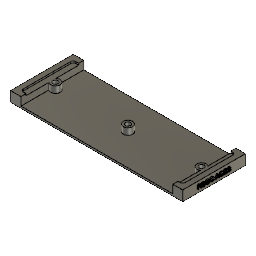
FullSizeHolder v4 (Autodesk Fusion 360 design; units mm, degrees)
Autodesk Fusion 360 part; units mm, degrees
sketch "Solid" plane through (0, 0, 0) normal (0, 0, 1) x (1, 0, 0)
  line L0 (83.5, -30.5) -> (-83.5, -30.5)
  line L1 (-83.5, -30.5) -> (-83.5, 30.5)
  line L2 (-83.5, 30.5) -> (83.5, 30.5)
  line L3 (83.5, 30.5) -> (83.5, -30.5)
  line L4 (83.5, -30.5) -> (-83.5, 30.5) construction
  line L5 (-83.5, -30.5) -> (83.5, 30.5) construction
  dimension "d13" = 167
  dimension "d14" = 61
  constraint horizontal L0
  constraint perpendicular L0 L1
  constraint parallel L0 L2
  constraint parallel L1 L3
  constraint coincident L4 origin
  constraint coincident L5 origin
  measures "d13" distance of L1.end L2.end
  measures "d14" distance of L0.end L1.end
extrude "Extrude1" add sketch "Solid" along normal blind 10
sketch "FR4Recess" plane through (0, 0, 10) normal (0, 0, 1) x (-1, 0, 0)
  line L0 (-83.5, -30.5) -> (83.5, -30.5)
  line L1 (83.5, -30.5) -> (83.5, 30.5)
  line L2 (83.5, 30.5) -> (-83.5, 30.5)
  line L3 (-83.5, 30.5) -> (-83.5, -30.5)
  line L4 (75.96, 25.5) -> (-75.96, 25.5)
  line L5 (-78.5, 22.96) -> (-78.5, -22.96)
  line L6 (-75.96, -25.5) -> (75.96, -25.5)
  line L7 (78.5, -22.96) -> (78.5, 22.96)
  line L8 (78.5, 25.5) -> (-78.5, -25.5) construction
  line L9 (-78.5, 25.5) -> (78.5, -25.5) construction
  arc A0 (75.96, -25.5) -> (78.5, -22.96) centre (75.96, -22.96) ccw
  arc A1 (78.5, 22.96) -> (75.96, 25.5) centre (75.96, 22.96) ccw
  arc A2 (-75.96, 25.5) -> (-78.5, 22.96) centre (-75.96, 22.96) ccw
  arc A3 (-78.5, -22.96) -> (-75.96, -25.5) centre (-75.96, -22.96) ccw
  dimension "d17" = 157
  dimension "d18" = 51
  dimension "d19" = 2.54
  dimension "d20" = 2.54
  dimension "d21" = 2.54
  dimension "d22" = 2.54
  constraint horizontal L4
  constraint perpendicular L4 L5
  constraint parallel L4 L6
  constraint parallel L5 L7
  constraint coincident L8 origin
  constraint coincident L9 origin
  constraint coincident L9.end L6
  constraint coincident L9.end L7
  constraint tangent L6 A0
  constraint tangent L7 A0
  constraint coincident L8.start L4
  constraint coincident L8.start L7
  constraint tangent L4 A1
  constraint tangent L7 A1
  constraint coincident L9.start L4
  constraint coincident L9.start L5
  constraint tangent L4 A2
  constraint tangent L5 A2
  constraint coincident L8.end L6
  constraint coincident L8.end L5
  constraint tangent L6 A3
  constraint tangent L5 A3
  measures "d17" distance of L8.end L9.end
  measures "d18" distance of L9.start L8.end
  measures "d19" radius of A0
  measures "d20" radius of A1
  measures "d21" radius of A2
  measures "d22" radius of A3
extrude "Extrude2" cut sketch "FR4Recess" against normal blind 1.68 contours L4 L5 L6 L7 A0 A1 A2 A3
sketch "Extrude" plane through (0, 0, 10) normal (0, 0, 1) x (-1, 0, 0)
  line L0 (73.2312, -31.7537) -> (-73.9375, -31.7537)
  line L1 (-73.9375, -31.7537) -> (-73.9375, 32.0704)
  line L2 (-73.9375, 32.0704) -> (73.2312, 32.0704)
  line L3 (73.2312, 32.0704) -> (73.2312, -31.7537)
  constraint horizontal L0
  constraint vertical L1
  constraint horizontal L2
  constraint vertical L3
extrude "Extrude6" cut sketch "Extrude" against normal blind 8
sketch "PierCenter" plane through (0, 0, 2) normal (0, 0, 1) x (-1, 0, 0)
  line L0 (73.2312, 30.5) -> (-73.9375, 30.5)
  line L1 (-73.9375, 30.5) -> (-73.9375, -30.5)
  line L2 (-73.9375, -30.5) -> (73.2312, -30.5)
  line L3 (73.2312, -30.5) -> (73.2312, 30.5)
  circle A0 centre (0, 0) radius 4.5
  circle A1 centre (0, 0) radius 2.5
  dimension "d33" = 9
  dimension "d34" = 5
  constraint coincident A0.centre A1.centre
  constraint concentric A0 A1
  measures "d33" diameter of A0
  measures "d34" diameter of A1
extrude "Extrude7" add sketch "PierCenter" along normal blind 6.32 contours A0
sketch "PierLeft" plane through (0, 0, 2) normal (0, 0, 1) x (-1, 0, 0)
  line L0 (73.2312, 30.5) -> (-73.9375, 30.5)
  line L1 (-73.9375, 30.5) -> (-73.9375, -30.5)
  line L2 (-73.9375, -30.5) -> (73.2312, -30.5)
  line L3 (73.2312, -30.5) -> (73.2312, 30.5)
  circle A0 centre (0, 0) radius 4.5
  circle A1 centre (70.3114, -0.0182) radius 4.5
  circle A2 centre (70.3114, -0.0182) radius 2.5
  point P0 (70.3114, -0.0182)
  dimension "d37" = 9
  dimension "d38" = 5
  constraint coincident P0 A1.centre
  measures "d37" diameter of A1
  measures "d38" diameter of A2
extrude "Extrude8" add sketch "PierLeft" along normal blind 6.32 contours L3 A1 picked at (66.4862, -0.0182)
sketch "PierRight" plane through (0, 0, 2) normal (0, 0, 1) x (-1, 0, 0)
  arc A0 (73.2312, 3.406) -> (73.2312, -3.4424) centre (70.3114, -0.0182) ccw
  line L0 (73.2312, 3.406) -> (73.2312, 30.5)
  line L1 (73.2312, 30.5) -> (-73.9375, 30.5)
  line L2 (-73.9375, 30.5) -> (-73.9375, -30.5)
  line L3 (-73.9375, -30.5) -> (73.2312, -30.5)
  line L4 (73.2312, -30.5) -> (73.2312, -3.4424)
  circle A1 centre (0, 0) radius 4.5
  circle A2 centre (-71.2906, 0.0558) radius 4.5
  circle A3 centre (-71.2906, 0.0558) radius 2.5
  point P0 (-71.2906, 0.0558)
  dimension "d41" = 9
  dimension "d42" = 5
  constraint coincident P0 A2.centre
  constraint concentric A2 A3
  measures "d41" diameter of A2
  measures "d42" diameter of A3
extrude "Extrude9" add sketch "PierRight" along normal blind 6.32 contours L2 A2 picked at (-73.2852, 3.3195)
sketch "RSGCACES" plane through (83.5, 0, 0) normal (1, 0, 0) x (0, 1, 0)
  line L0 (-30.5, 0) -> (30.5, 0)
  line L1 (30.5, 0) -> (30.5, 10)
  line L2 (30.5, 10) -> (-30.5, 10)
  line L3 (-30.5, 10) -> (-30.5, 0)
  line L4 (-18.8418, 2.2772) -> (17.8909, 2.2772) construction
  line L5 (17.8909, 2.2772) -> (17.8909, 8.5407) construction
  line L6 (17.8909, 8.5407) -> (-18.8418, 8.5407) construction
  line L7 (-18.8418, 8.5407) -> (-18.8418, 2.2772) construction
  dimension "d45" = 4
  text T0 "RSGC ACES" font "Arial" height 4 align centre middle in box 36.7327 x 6.2635 at (-18.8418, 2.2772) x (1, 0) y (0, 1) spacing 1 kerned
extrude "Extrude10" add sketch "RSGCACES" along normal blind 1 text T0
sketch "PermaProto" plane through (-83.5, 0, 0) normal (-1, 0, 0) x (0, -1, 0)
  line L0 (-30.5, 0) -> (30.5, 0)
  line L1 (30.5, 0) -> (30.5, 10)
  line L2 (30.5, 10) -> (-30.5, 10)
  line L3 (-30.5, 10) -> (-30.5, 0)
  line L4 (-23.5941, 1.9572) -> (24.0905, 1.9572) construction
  line L5 (24.0905, 1.9572) -> (24.0905, 8.5295) construction
  line L6 (24.0905, 8.5295) -> (-23.5941, 8.5295) construction
  line L7 (-23.5941, 8.5295) -> (-23.5941, 1.9572) construction
  dimension "d48" = 4
  text T0 "Perma-Proto" font "Arial" height 4 align centre middle in box 47.6846 x 6.5724 at (-23.5941, 1.9572) x (1, 0) y (0, 1) spacing 1 kerned
extrude "Extrude11" add sketch "PermaProto" along normal blind 1 text T0
sketch "ACESLogo" plane through (0, 0, 0) normal (0, 0, 1) x (1, 0, 0)
  arc A0 (-0.5552, -1.4875) -> (-1.5641, -1.6462) centre (-1.6183, 1.9835) cw
  spline S0 degree 3 poles (-1.5641, -1.6462) (-2.3665, -1.5998) (-3.0241, -0.9925) (-3.134, -0.1963) knots 1 1 1 1 2 2 2 2
  arc A1 (-3.134, -0.1963) -> (-2.6789, 1.1936) centre (-1.2347, -0.0487) cw
  spline S1 degree 3 poles (-2.6789, 1.1936) (-1.9451, 2.0932) (-1.2008, 2.9857) (-0.467, 3.8889) knots 3 3 3 3 4 4 4 4
  spline S2 degree 3 poles (-0.467, 3.8889) (-0.307, 4.097) (-0.0088, 4.1364) (0.1997, 3.9771) knots 4 4 4 4 5 5 5 5
  arc A2 (0.1997, 3.9771) -> (0.2879, 3.8889) centre (-0.0472, 3.6419) cw
  spline S3 degree 3 poles (0.2879, 3.8889) (0.7289, 3.3279) (1.1981, 2.7952) (1.6497, 2.2449) knots 6 6 6 6 7 7 7 7
  arc A3 (1.6497, 2.2449) -> (2.6657, 0.982) centre (-8.6979, -7.1195) cw
  spline S4 degree 3 poles (2.6657, 0.982) (3.195, 0.2422) (3.0262, -0.7863) (2.2882, -1.3181) knots 8 8 8 8 9 9 9 9
  arc A4 (2.2882, -1.3181) -> (1.7026, -1.5827) centre (1.3109, 0.0647) cw
  arc A5 (1.7026, -1.5827) -> (0.5702, -1.5263) centre (1.2508, 0.7409) cw
  spline S5 degree 3 poles (0.5702, -1.5263) (0.5067, -1.5263) (0.422, -1.4451) (0.3373, -1.551) (0.4044, -1.6251) (0.4255, -1.6886) knots 11 11 11 11 12 12 13 13 13 13
  arc A6 (0.4255, -1.6886) -> (0.7889, -2.3341) centre (4.0074, -0.0976) ccw
  spline S6 degree 3 poles (0.7889, -2.3341) (0.8348, -2.4047) (0.8947, -2.4788) (0.7889, -2.6622) (0.7007, -2.6446) (0.6125, -2.6446) knots 14 14 14 14 15 15 16 16 16 16
  line L0 (0.6125, -2.6446) -> (-0.7986, -2.6446)
  arc A7 (-0.7986, -2.6446) -> (-0.9785, -2.5634) centre (-0.8165, -2.4443) cw
  spline S7 degree 3 poles (-0.9785, -2.5634) (-1.0279, -2.4894) (-0.9785, -2.4294) (-0.9503, -2.3694) knots 18 18 18 18 19 19 19 19
  arc A8 (-0.9503, -2.3694) -> (-0.5552, -1.4875) centre (-3.2707, -0.8004) ccw
  arc A9 (0.362, -5.6326) -> (0.7501, -6.4899) centre (3.1563, -4.8842) ccw
  arc A10 (0.7501, -6.4899) -> (0.8171, -6.5886) centre (-0.0176, -7.0829) cw
  spline S8 degree 3 poles (0.8171, -6.5886) (0.8585, -6.657) (0.8367, -6.7459) (0.7684, -6.7873) knots 2 2 2 2 3 3 3 3
  spline S9 degree 3 poles (0.7684, -6.7873) (0.767, -6.7881) (0.7656, -6.7889) (0.7642, -6.7897) knots 3 3 3 3 4 4 4 4
  arc A11 (0.7642, -6.7897) -> (0.6795, -6.8109) centre (0.6938, -6.6882) cw
  line L1 (0.6795, -6.8109) -> (-0.8692, -6.8109)
  spline S10 degree 3 poles (-0.8692, -6.8109) (-1.0138, -6.8109) (-1.0703, -6.698) (-0.9926, -6.571) knots 6 6 6 6 7 7 7 7
  arc A12 (-0.9926, -6.571) -> (-0.5975, -5.7984) centre (-4.0766, -4.5065) ccw
  spline S11 degree 3 poles (-0.5975, -5.7984) (-0.5799, -5.749) (-0.5481, -5.6926) (-0.6469, -5.622) (-0.6787, -5.6573) (-0.721, -5.6785) knots 8 8 8 8 9 9 10 10 10 10
  arc A13 (-0.721, -5.6785) -> (-2.1533, -5.6573) centre (-1.4054, -3.5232) cw
  spline S12 degree 3 poles (-2.1533, -5.6573) (-2.7471, -5.4029) (-3.1374, -4.825) (-3.1516, -4.1792) knots 11 11 11 11 12 12 12 12
  arc A14 (-3.1516, -4.1792) -> (-3.0917, -3.6923) centre (-1.2679, -4.1641) cw
  spline S13 degree 3 poles (-3.0917, -3.6923) (-3.0773, -3.6102) (-3.0018, -3.5531) (-2.9188, -3.5618) knots 13 13 13 13 14 14 14 14
  line L2 (-2.9188, -3.5618) -> (2.6445, -3.5618)
  spline S14 degree 3 poles (2.6445, -3.5618) (2.8032, -3.5618) (2.8738, -3.6147) (2.9056, -3.7594) knots 15 15 15 15 16 16 16 16
  spline S15 degree 3 poles (2.9056, -3.7594) (3.1249, -4.6304) (2.5966, -5.5142) (1.7256, -5.7336) knots 16 16 16 16 17 17 17 17
  line L3 (1.7256, -5.7336) -> (1.7202, -5.7349)
  line L4 (1.7202, -5.7349) -> (1.6673, -5.7349)
  arc A15 (1.6673, -5.7349) -> (0.362, -5.6326) centre (1.2187, -3.0809) cw
  spline S16 degree 3 poles (-4.9861, -1.4875) (-5.2154, -1.5439) (-5.4341, -1.5898) (-5.6528, -1.6251) knots 0 0 0 0 1 1 1 1
  spline S17 degree 3 poles (-5.6528, -1.6251) (-6.5586, -1.7725) (-7.4123, -1.1577) (-7.5598, -0.252) (-7.6373, 0.2242) (-7.5039, 0.7106) (-7.1945, 1.0808) knots 1 1 1 1 2 2 2 3 3 3 3
  spline S18 degree 3 poles (-7.1945, 1.0808) (-6.7606, 1.6417) (-6.2984, 2.1779) (-5.8539, 2.7247) knots 3 3 3 3 4 4 4 4
  line L5 (-5.8539, 2.7247) -> (-4.8944, 3.8959)
  arc A16 (-4.8944, 3.8959) -> (-4.5416, 4.0723) centre (-4.5522, 3.6526) cw
  spline S19 degree 3 poles (-4.5416, 4.0723) (-4.454, 4.0763) (-4.3798, 4.0085) (-4.3758, 3.9209) knots 6 6 6 6 7 7 7 7
  line L6 (-4.3758, 3.9209) -> (-4.3758, 3.9206)
  line L7 (-4.3758, 3.9206) -> (-4.3758, -2.4858)
  spline S20 degree 3 poles (-4.3758, -2.4858) (-4.356, -2.5763) (-4.4126, -2.6659) (-4.5028, -2.6869) knots 9 9 9 9 10 10 10 10
  line L8 (-4.5028, -2.6869) -> (-5.2577, -2.6869)
  arc A17 (-5.2577, -2.6869) -> (-5.4482, -2.5917) centre (-5.2823, -2.498) cw
  spline S21 degree 3 poles (-5.4482, -2.5917) (-5.4941, -2.5246) (-5.4482, -2.4682) (-5.4129, -2.4153) knots 12 12 12 12 13 13 13 13
  arc A18 (-5.4129, -2.4153) -> (-4.9861, -1.4875) centre (-7.9879, -0.6685) ccw
  line L9 (4.2002, 0.7068) -> (4.2002, 3.8077)
  spline S22 degree 3 poles (4.2002, 3.8077) (4.2002, 3.8994) (4.1614, 4.0159) (4.2814, 4.0582) knots 1 1 1 1 2 2 2 2
  arc A19 (4.2814, 4.0582) -> (4.6059, 3.9876) centre (4.3827, 3.7424) cw
  arc A20 (4.6059, 3.9876) -> (4.9305, 3.6102) centre (2.8461, 2.1463) cw
  spline S23 degree 3 poles (4.9305, 3.6102) (5.6184, 2.7811) (6.3169, 1.9556) (6.9837, 1.109) knots 4 4 4 4 5 5 5 5
  spline S24 degree 3 poles (6.9837, 1.109) (7.5909, 0.4209) (7.5253, -0.6291) (6.8372, -1.2363) (6.4609, -1.5684) (5.9545, -1.7126) (5.4597, -1.6286) knots 5 5 5 5 6 6 6 7 7 7 7
  spline S25 degree 3 poles (5.4597, -1.6286) (5.2692, -1.6004) (5.0857, -1.5686) (4.8988, -1.5228) knots 7 7 7 7 8 8 8 8
  spline S26 degree 3 poles (4.8988, -1.5228) (4.8705, -1.5228) (4.8458, -1.4839) (4.7894, -1.5616) (4.8176, -1.5757) (4.8176, -1.6074) knots 8 8 8 8 9 9 10 10 10 10
  arc A21 (4.8176, -1.6074) -> (5.1457, -2.313) centre (7.942, -0.5836) ccw
  spline S27 degree 3 poles (5.1457, -2.313) (5.2021, -2.4118) (5.315, -2.5035) (5.181, -2.7504) (5.0399, -2.6975) (4.9305, -2.701) knots 11 11 11 11 12 12 13 13 13 13
  line L10 (4.9305, -2.701) -> (4.4013, -2.701)
  spline S28 degree 3 poles (4.4013, -2.701) (4.2249, -2.701) (4.1967, -2.6658) (4.1967, -2.4999) knots 14 14 14 14 15 15 15 15
  line L11 (4.1967, -2.4999) -> (4.2002, 0.7068)
  line L12 (2.3023, 5.0036) -> (0.9723, 5.0036)
  spline S29 degree 3 poles (0.9723, 5.0036) (0.4679, 5.0036) (-0.0401, 4.9789) (-0.5446, 5.0036) knots 1 1 1 1 2 2 2 2
  line L13 (-0.5446, 5.0036) -> (-2.6048, 5.0036)
  arc A22 (-2.6048, 5.0036) -> (-2.7777, 5.0918) centre (-2.6224, 5.1827) cw
  ellipse E0 centre (-2.6432, 5.157) end of major axis (-2.6115, 5.304) minor radius 0.1488 (-2.7389, 5.2717) -> (-2.7777, 5.0918) ccw
  arc A23 (-2.7389, 5.2717) -> (-0.467, 8.0305) centre (494.7406, -402.1025) cw
  spline S30 degree 3 poles (-0.467, 8.0305) (-0.3293, 8.2375) (-0.0502, 8.2943) (0.1574, 8.1575) knots 6 6 6 6 7 7 7 7
  arc A24 (0.1574, 8.1575) -> (0.2985, 8.0093) centre (-0.08, 7.7901) cw
  spline S31 degree 3 poles (0.2985, 8.0093) (0.6125, 7.6177) (0.9406, 7.2367) (1.2616, 6.8487) knots 8 8 8 8 9 9 9 9
  line L14 (1.2616, 6.8487) -> (2.3199, 5.554)
  spline S32 degree 3 poles (2.3199, 5.554) (2.3976, 5.4587) (2.4716, 5.3635) (2.5528, 5.2753) knots 10 10 10 10 11 11 11 11
  ellipse E1 centre (2.4602, 5.1624) end of major axis (2.4286, 5.3059) minor radius 0.1453 (2.5916, 5.0989) -> (2.5528, 5.2753) ccw
  spline S33 degree 3 poles (2.5916, 5.0989) (2.5643, 5.0318) (2.4934, 4.9934) (2.4223, 5.0072) knots 12 12 12 12 13 13 13 13
  arc A25 (2.4223, 5.0072) -> (2.3023, 5.0036) centre (2.3725, 4.6579) ccw
  arc A26 (4.8423, -5.6397) -> (5.248, -6.5004) centre (7.9138, -4.718) ccw
  spline S34 degree 3 poles (5.248, -6.5004) (5.2903, -6.5675) (5.3397, -6.631) (5.248, -6.8074) (5.1669, -6.7862) (5.0963, -6.7862) knots 1 1 1 1 2 2 3 3 3 3
  line L15 (5.0963, -6.7862) -> (4.419, -6.7862)
  spline S35 degree 3 poles (4.419, -6.7862) (4.2849, -6.7862) (4.232, -6.7297) (4.232, -6.5957) knots 4 4 4 4 5 5 5 5
  line L16 (4.232, -6.5957) -> (4.232, -3.7453)
  spline S36 degree 3 poles (4.232, -3.7453) (4.232, -3.6147) (4.2884, -3.5477) (4.419, -3.5477) knots 6 6 6 6 7 7 7 7
  line L17 (4.419, -3.5477) -> (7.1848, -3.5477)
  spline S37 degree 3 poles (7.1848, -3.5477) (7.2676, -3.5364) (7.3454, -3.5898) (7.3647, -3.6712) knots 8 8 8 8 9 9 9 9
  spline S38 degree 3 poles (7.3647, -3.6712) (7.6112, -4.543) (7.1043, -5.4495) (6.2325, -5.696) knots 9 9 9 9 10 10 10 10
  line L18 (6.2325, -5.696) -> (6.2323, -5.6961)
  arc A27 (6.2323, -5.6961) -> (6.0029, -5.742) centre (5.7724, -3.9931) cw
  arc A28 (6.0029, -5.742) -> (4.9446, -5.622) centre (5.7859, -2.9281) cw
  line L19 (4.9446, -5.622) -> (4.8846, -5.622)
  line L20 (4.8846, -5.622) -> (4.8423, -5.6397)
  arc A29 (-4.9896, -5.6361) -> (-5.9774, -5.7808) centre (-6.0199, -2.0451) cw
  spline S39 degree 3 poles (-5.9774, -5.7808) (-6.5657, -5.7727) (-7.1045, -5.4494) (-7.3885, -4.9341) knots 1 1 1 1 2 2 2 2
  arc A30 (-7.3885, -4.9341) -> (-7.5331, -3.7453) centre (-6.0354, -4.1663) cw
  spline S40 degree 3 poles (-7.5331, -3.7453) (-7.5138, -3.6474) (-7.4245, -3.5793) (-7.325, -3.5865) knots 3 3 3 3 4 4 4 4
  line L21 (-7.325, -3.5865) -> (-4.6051, -3.5865)
  spline S41 degree 3 poles (-4.6051, -3.5865) (-4.4252, -3.5865) (-4.3934, -3.6253) (-4.3934, -3.8123) knots 5 5 5 5 6 6 6 6
  line L22 (-4.3934, -3.8123) -> (-4.3934, -6.6027)
  spline S42 degree 3 poles (-4.3934, -6.6027) (-4.3934, -6.7544) (-4.4428, -6.8109) (-4.598, -6.8109) knots 7 7 7 7 8 8 8 8
  line L23 (-4.598, -6.8109) -> (-5.2507, -6.8109)
  arc A31 (-5.2507, -6.8109) -> (-5.4482, -6.7297) centre (-5.2863, -6.6166) cw
  spline S43 degree 3 poles (-5.4482, -6.7297) (-5.4976, -6.6486) (-5.4482, -6.5957) (-5.4094, -6.5357) knots 10 10 10 10 11 11 11 11
  arc A32 (-5.4094, -6.5357) -> (-4.9896, -5.6361) centre (-7.8372, -4.855) ccw
  line L24 (4.2285, 6.5982) -> (4.2285, 8.0093)
  spline S44 degree 3 poles (4.2285, 8.0093) (4.2285, 8.1963) (4.3167, 8.2739) (4.5248, 8.2139) knots 1 1 1 1 2 2 2 2
  arc A33 (4.5248, 8.2139) -> (4.7329, 8.0728) centre (4.402, 7.8088) cw
  line L25 (4.7329, 8.0728) -> (5.7913, 6.7746)
  line L26 (5.7913, 6.7746) -> (6.9696, 5.3635)
  arc A34 (6.9696, 5.3635) -> (7.0613, 5.2435) centre (6.5428, 4.9421) cw
  spline S45 degree 3 poles (7.0613, 5.2435) (7.1007, 5.1832) (7.0837, 5.1023) (7.0234, 5.0629) knots 6 6 6 6 7 7 7 7
  ellipse E2 centre (6.9292, 5.1661) end of major axis (7.0726, 5.1299) minor radius 0.1252 (7.0189, 5.0601) -> (7.0234, 5.0629) ccw
  arc A35 (7.0189, 5.0601) -> (6.9449, 5.0389) centre (6.9426, 5.1871) cw
  line L27 (6.9449, 5.0389) -> (4.3625, 5.0389)
  spline S46 degree 3 poles (4.3625, 5.0389) (4.2355, 5.0389) (4.2249, 5.1271) (4.2249, 5.2259) knots 10 10 10 10 11 11 11 11
  line L28 (4.2249, 5.2259) -> (4.2249, 6.5982)
  line L29 (4.2249, 6.5982) -> (4.2285, 6.5982)
  spline S47 degree 3 poles (-4.404, 6.958) (-4.3722, 6.5559) (-4.4216, 6.0796) (-4.3828, 5.6069) knots 0 0 0 0 1 1 1 1
  line L30 (-4.3828, 5.6069) -> (-4.3828, 5.1589)
  spline S48 degree 3 poles (-4.3828, 5.1589) (-4.3768, 5.0753) (-4.4396, 5.0027) (-4.5232, 4.9966) knots 2 2 2 2 3 3 3 3
  line L31 (-4.5232, 4.9966) -> (-4.5239, 4.9966)
  line L32 (-4.5239, 4.9966) -> (-6.1326, 4.9966)
  line L33 (-6.1326, 4.9966) -> (-7.0851, 4.9966)
  spline S49 degree 3 poles (-7.0851, 4.9966) (-7.1607, 4.9884) (-7.2285, 5.0431) (-7.2367, 5.1186) knots 6 6 6 6 7 7 7 7
  line L34 (-7.2367, 5.1186) -> (-7.2368, 5.1201)
  arc A36 (-7.2368, 5.1201) -> (-7.1909, 5.2365) centre (-7.0925, 5.1305) cw
  spline S50 degree 3 poles (-7.1909, 5.2365) (-6.8382, 5.6633) (-6.4854, 6.0902) (-6.1326, 6.51) knots 9 9 9 9 10 10 10 10
  line L35 (-6.1326, 6.51) -> (-5.2083, 7.6989)
  spline S51 degree 3 poles (-5.2083, 7.6989) (-5.106, 7.8259) (-5.0002, 7.9564) (-4.8944, 8.0799) knots 11 11 11 11 12 12 12 12
  arc A37 (-4.8944, 8.0799) -> (-4.591, 8.221) centre (-4.5754, 7.7909) cw
  spline S52 degree 3 poles (-4.591, 8.221) (-4.5059, 8.2316) (-4.4283, 8.1713) (-4.4177, 8.0862) (-4.416, 8.0724) (-4.4161, 8.0584) (-4.4181, 8.0446) knots 13 13 13 13 14 14 14 15 15 15 15
  spline S53 degree 3 poles (-4.4181, 8.0446) (-4.4075, 7.7059) (-4.404, 7.3672) (-4.404, 6.958) knots 15 15 15 15 16 16 16 16
  line L36 (8.2784, 0.1565) -> (8.2784, 1.6276)
  spline S54 degree 3 poles (8.2784, 1.6276) (8.2784, 1.7087) (8.2784, 1.7863) (8.3666, 1.8181) knots 1 1 1 1 2 2 2 2
  spline S55 degree 3 poles (8.3666, 1.8181) (8.4344, 1.8499) (8.5153, 1.8274) (8.5571, 1.7651) knots 2 2 2 2 3 3 3 3
  spline S56 degree 3 poles (8.5571, 1.7651) (8.7617, 1.4935) (9.0121, 1.2536) (9.1921, 0.9608) knots 3 3 3 3 4 4 4 4
  spline S57 degree 3 poles (9.1921, 0.9608) (9.5878, 0.3976) (9.5962, -0.3511) (9.2132, -0.923) knots 4 4 4 4 5 5 5 5
  arc A38 (9.2132, -0.923) -> (8.55, -1.4804) centre (7.7815, 0.1073) cw
  spline S58 degree 3 poles (8.55, -1.4804) (8.3736, -1.5721) (8.2713, -1.5016) (8.2713, -1.3005) knots 6 6 6 6 7 7 7 7
  line L37 (8.2713, -1.3005) -> (8.2713, 0.1565)
  line L38 (8.2713, 0.1565) -> (8.2784, 0.1565)
  line L39 (-8.4786, 0.1353) -> (-8.4786, -1.3111)
  ellipse E3 centre (-9.7979, 0.5867) end of major axis (-11.0461, 2.6795) minor radius 0.4973 (-8.7467, -1.4804) -> (-8.4786, -1.3111) ccw
  spline S59 degree 3 poles (-8.7467, -1.4804) (-9.2238, -1.2603) (-9.5645, -0.8223) (-9.6604, -0.3057) knots 2 2 2 2 3 3 3 3
  ellipse E4 centre (-7.9359, -0.0084) end of major axis (-7.4669, 1.6844) minor radius 1.7485 (-9.2617, 1.1337) -> (-9.6604, -0.3057) ccw
  spline S60 degree 3 poles (-9.2617, 1.1337) (-9.0889, 1.3489) (-8.9196, 1.5464) (-8.7361, 1.7722) knots 4 4 4 4 5 5 5 5
  ellipse E5 centre (-8.6173, 1.6875) end of major axis (-8.4758, 1.7271) minor radius 0.1453 (-8.5597, 1.8216) -> (-8.7361, 1.7722) ccw
  spline S61 degree 3 poles (-8.5597, 1.8216) (-8.4821, 1.7934) (-8.4645, 1.7334) (-8.4645, 1.6558) knots 6 6 6 6 7 7 7 7
  spline S62 degree 3 poles (-8.4645, 1.6558) (-8.4821, 1.1513) (-8.4786, 0.6504) (-8.4786, 0.1353) knots 7 7 7 7 8 8 8 8
  line L40 (-0.1036, 9.0888) -> (-1.162, 9.0888)
  spline S63 degree 3 poles (-1.162, 9.0888) (-1.2431, 9.0888) (-1.3137, 9.0888) (-1.3913, 9.2723) (-1.3525, 9.3146) (-1.296, 9.371) knots 1 1 1 1 2 2 3 3 3 3
  line L41 (-1.296, 9.371) -> (-0.4353, 10.4294)
  spline S64 degree 3 poles (-0.4353, 10.4294) (-0.2676, 10.6162) (0.0197, 10.632) (0.2068, 10.4646) knots 4 4 4 4 5 5 5 5
  ellipse E6 centre (-0.0094, 10.2133) end of major axis (0.3199, 10.1741) minor radius 0.3315 (0.2421, 10.4294) -> (0.2068, 10.4646) ccw
  spline S65 degree 3 poles (0.2421, 10.4294) (0.5419, 10.0766) (0.8277, 9.7238) (1.1205, 9.3534) knots 6 6 6 6 7 7 7 7
  spline S66 degree 3 poles (1.1205, 9.3534) (1.1664, 9.3005) (1.2157, 9.2476) (1.1699, 9.1664) knots 7 7 7 7 8 8 8 8
  ellipse E7 centre (1.0127, 9.2561) end of major axis (1.178, 9.3325) minor radius 0.1804 (0.9794, 9.0782) -> (1.1699, 9.1664) ccw
  line L42 (0.9794, 9.0782) -> (-0.1036, 9.0888)
  line L43 (-0.086, -9.1569) -> (-0.8586, -9.1569)
  arc A39 (-0.8586, -9.1569) -> (-1.0138, -9.0863) centre (-0.8843, -9.0074) cw
  arc A40 (-1.0138, -9.0863) -> (-0.9891, -8.9029) centre (-0.8568, -9.0141) cw
  arc A41 (-0.9891, -8.9029) -> (-0.5587, -8.0068) centre (-3.2975, -7.2427) ccw
  line L44 (-0.5587, -8.0068) -> (-0.5587, -7.9786)
  spline S67 degree 3 poles (-0.5587, -7.9786) (-0.4882, -7.6258) (-0.4882, -7.6258) (-0.1424, -7.6258) knots 5 5 5 5 6 6 6 6
  line L45 (-0.1424, -7.6258) -> (0.1292, -7.6258)
  spline S68 degree 3 poles (0.1292, -7.6258) (0.2167, -7.6108) (0.3001, -7.669) (0.3162, -7.7563) knots 7 7 7 7 8 8 8 8
  ellipse E8 centre (0.2718, -7.7669) end of major axis (0.2718, -7.7212) minor radius 0.0456 (0.3162, -7.7775) -> (0.3162, -7.7563) ccw
  arc A42 (0.3162, -7.7775) -> (0.7889, -8.8711) centre (2.642, -7.4211) ccw
  arc A43 (0.7889, -8.8711) -> (0.8277, -9.0969) centre (0.6045, -9.019) cw
  spline S69 degree 3 poles (0.8277, -9.0969) (0.7959, -9.171) (0.7113, -9.1569) (0.6407, -9.1569) knots 11 11 11 11 12 12 12 12
  line L46 (0.6407, -9.1569) -> (-0.086, -9.1569)
extrude "Extrude15" cut sketch "ACESLogo" along normal blind 1
extrude "Extrude16" cut sketch "PierCenter" against normal blind 0.78 contours A1
extrude "Extrude17" cut sketch "PierRight" against normal blind 0.68 contours A3
extrude "Extrude18" cut sketch "PierLeft" against normal blind 0.68 contours A2
extrude "Extrude4" [suppressed]
